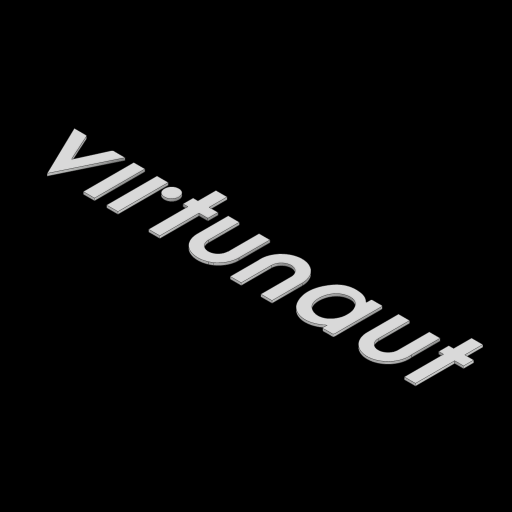
# Autodesk Inventor part: 242_LOGO
Saved by Autodesk Inventor 2024 (Build 280153000, 153)
## iProperties
Created: 2023-07-24
Part Number: 242_LOGO
Material: Generisch
Document SubType Name: Modeling
Designer: Philipp
Density: 1 g/cm^3
Appearance: Vorgabe
Author: Philipp
Autodesk Inventor part; units mm, degrees
ref_plane "YZ Plane" through (0, 0, 0) normal (1, 0, 0) x (0, 1, 0)
ref_plane "XZ Plane" through (0, 0, 0) normal (0, 1, 0) x (-1, 0, 0)
ref_plane "XY Plane" through (0, 0, 0) normal (0, 0, 1) x (1, 0, 0)
sketch "Skizze1" plane through (0, 0, 0) normal (0, 0, 1) x (1, 0, 0)
  line L0 (-37.3972, 3.9318) -> (-43.7451, -9.2055)
  line L1 (-43.7451, -9.2055) -> (-50.0897, 3.9182)
  line L2 (-32.4911, 3.9572) -> (-35.2833, 3.9572)
  line L3 (-35.2833, 3.9572) -> (-35.2833, -8.635)
  line L4 (-35.2833, -8.635) -> (-32.4911, -8.635)
  line L5 (-32.4911, -8.635) -> (-32.4911, 3.9572)
  line L6 (-26.6443, 3.9432) -> (-29.4671, 3.9432)
  line L7 (-29.4671, 3.9432) -> (-29.4671, -8.635)
  line L8 (-29.4671, -8.635) -> (-26.6443, -8.635)
  line L9 (-26.6443, -8.635) -> (-26.6443, 3.9432)
  line L10 (-16.1812, 3.676) -> (-16.1812, 8.1673)
  line L11 (-16.1812, 8.1673) -> (-18.9705, 8.1673)
  line L12 (-18.9705, 8.1673) -> (-18.9705, 3.676)
  line L13 (-18.9705, 3.676) -> (-20.1816, 3.676)
  line L14 (-20.1816, 3.676) -> (-20.1816, 1.149)
  line L15 (-20.1816, 1.149) -> (-18.9705, 1.149)
  line L16 (-18.9705, 1.149) -> (-18.9705, -8.635)
  line L17 (-18.9705, -8.635) -> (-16.1812, -8.635)
  line L18 (-16.1812, -8.635) -> (-16.1812, 1.149)
  line L19 (-16.1812, 1.149) -> (-13.9526, 1.149)
  line L20 (-13.9526, 1.149) -> (-13.9526, 3.676)
  line L21 (-13.9526, 3.676) -> (-16.1812, 3.676)
  arc A0 (-3.6373, -7.7101) -> (-1.5254, -3.5201) centre (-6.7378, -3.5201) ccw
  line L22 (-1.5254, -3.5201) -> (-1.5254, 4.2241)
  line L23 (-1.5254, 4.2241) -> (-4.2557, 4.2241)
  line L24 (-4.2557, 4.2241) -> (-4.2557, -3.5201)
  line L25 (-4.2557, -3.5201) -> (-4.3028, -3.5201)
  arc A1 (-9.1728, -3.5201) -> (-4.3028, -3.5201) centre (-6.7378, -3.5201) ccw
  line L26 (-9.1728, -3.5201) -> (-9.1728, 4.2241)
  line L27 (-9.1728, 4.2241) -> (-11.9502, 4.2241)
  line L28 (-11.9502, 4.2241) -> (-11.9502, -3.5201)
  arc A2 (-11.9502, -3.5201) -> (-10.9081, -6.647) centre (-6.7378, -3.5201) ccw
  line L29 (1.4099, -8.6315) -> (4.1527, -8.6315)
  line L30 (4.1527, -8.6315) -> (4.1527, -1.0852)
  arc A3 (9.0698, -1.0852) -> (4.1527, -1.0852) centre (6.6113, -1.0852) ccw
  line L31 (9.0698, -1.0852) -> (9.0698, -8.6315)
  line L32 (9.0698, -8.6315) -> (11.8472, -8.6315)
  line L33 (11.8472, -8.6315) -> (11.8472, -1.0852)
  arc A4 (11.8472, -1.0852) -> (1.4099, -1.6856) centre (6.6113, -1.0852) ccw
  line L34 (1.4099, -1.6856) -> (1.4099, -8.6315)
  line L35 (33.3608, 4.2241) -> (30.5834, 4.2241)
  line L36 (30.5834, 4.2241) -> (30.5834, -3.6173)
  arc A5 (30.5834, -3.6173) -> (41.0081, -2.916) centre (35.8193, -3.6173) ccw
  line L37 (41.0081, -2.916) -> (41.0081, 4.2241)
  line L38 (41.0081, 4.2241) -> (38.2779, 4.2241)
  line L39 (38.2779, 4.2241) -> (38.2779, -3.6173)
  arc A6 (33.3608, -3.6173) -> (38.2779, -3.6173) centre (35.8193, -3.6173) ccw
  line L40 (33.3608, -3.6173) -> (33.3608, 4.2241)
  line L41 (47.6817, 3.676) -> (47.6817, 8.1673)
  line L42 (47.6817, 8.1673) -> (44.8924, 8.1673)
  line L43 (44.8924, 8.1673) -> (44.8924, 3.676)
  line L44 (44.8924, 3.676) -> (43.6812, 3.676)
  line L45 (43.6812, 3.676) -> (43.6812, 1.149)
  line L46 (43.6812, 1.149) -> (44.8924, 1.149)
  line L47 (44.8924, 1.149) -> (44.8924, -8.635)
  line L48 (44.8924, -8.635) -> (47.6817, -8.635)
  line L49 (47.6817, -8.635) -> (47.6817, 1.149)
  line L50 (47.6817, 1.149) -> (49.9103, 1.149)
  line L51 (49.9103, 1.149) -> (49.9103, 3.676)
  line L52 (49.9103, 3.676) -> (47.6817, 3.676)
  spline S0 degree 3 poles (-50.0897, 3.9182) (-49.0082, 3.9182) (-48.0657, 3.9279) (-47.124, 3.9049) (-47.0171, 3.9023) (-46.8727, 3.7347) (-46.8166, 3.6114) (-45.8869, 1.5682) (-44.9691, -0.4805) (-44.0466, -2.527) (-43.9721, -2.6922) (-43.8826, -2.8505) (-43.7495, -3.1111) knots -10 -10 -10 -10 -9 -9 -9 -8 -8 -8 -7 -7 -7 -6 -6 -6 -6
  line L53 (-50.0897, 3.9182) -> (-49.0082, 3.9182) construction
  line L54 (-49.0082, 3.9182) -> (-48.0657, 3.9279) construction
  line L55 (-48.0657, 3.9279) -> (-47.124, 3.9049) construction
  line L56 (-47.124, 3.9049) -> (-47.0171, 3.9023) construction
  line L57 (-47.0171, 3.9023) -> (-46.8727, 3.7347) construction
  line L58 (-46.8727, 3.7347) -> (-46.8166, 3.6114) construction
  line L59 (-46.8166, 3.6114) -> (-45.8869, 1.5682) construction
  line L60 (-45.8869, 1.5682) -> (-44.9691, -0.4805) construction
  line L61 (-44.9691, -0.4805) -> (-44.0466, -2.527) construction
  line L62 (-44.0466, -2.527) -> (-43.9721, -2.6922) construction
  line L63 (-43.9721, -2.6922) -> (-43.8826, -2.8505) construction
  line L64 (-43.8826, -2.8505) -> (-43.7495, -3.1111) construction
  spline S1 degree 3 poles (-43.7495, -3.1111) (-43.6007, -2.8191) (-43.4873, -2.6166) (-43.3918, -2.406) (-42.4883, -0.4134) (-41.5817, 1.5779) (-40.6937, 3.5774) (-40.5751, 3.8444) (-40.4324, 3.9417) (-40.1479, 3.937) (-39.2783, 3.9226) (-38.4083, 3.9318) (-37.3972, 3.9318) knots -6 -6 -6 -6 -5 -5 -5 -4 -4 -4 -3 -3 -3 -2 -2 -2 -2
  line L65 (-43.7495, -3.1111) -> (-43.6007, -2.8191) construction
  line L66 (-43.6007, -2.8191) -> (-43.4873, -2.6166) construction
  line L67 (-43.4873, -2.6166) -> (-43.3918, -2.406) construction
  line L68 (-43.3918, -2.406) -> (-42.4883, -0.4134) construction
  line L69 (-42.4883, -0.4134) -> (-41.5817, 1.5779) construction
  line L70 (-41.5817, 1.5779) -> (-40.6937, 3.5774) construction
  line L71 (-40.6937, 3.5774) -> (-40.5751, 3.8444) construction
  line L72 (-40.5751, 3.8444) -> (-40.4324, 3.9417) construction
  line L73 (-40.4324, 3.9417) -> (-40.1479, 3.937) construction
  line L74 (-40.1479, 3.937) -> (-39.2783, 3.9226) construction
  line L75 (-39.2783, 3.9226) -> (-38.4083, 3.9318) construction
  line L76 (-38.4083, 3.9318) -> (-37.3972, 3.9318) construction
  line L77 (-35.2833, -8.635) -> (-35.2833, 3.9572)
  line L78 (-32.4911, 3.9572) -> (-32.4911, -8.635)
  spline S2 degree 3 poles (-25.7998, 2.1249) (-25.8047, 3.186) (-25.0538, 3.9433) (-23.9969, 3.9432) (-22.9712, 3.9431) (-22.2131, 3.1845) (-22.2062, 2.1515) (-22.199, 1.0897) (-22.9481, 0.3376) (-24.0112, 0.339) (-25.0478, 0.3403) (-25.7949, 1.0863) (-25.7998, 2.1249) knots -4 -4 -4 -4 -3 -3 -3 -2 -2 -2 -1 -1 -1 0 0 0 0
  line L79 (-25.7998, 2.1249) -> (-25.8047, 3.186) construction
  line L80 (-25.8047, 3.186) -> (-25.0538, 3.9433) construction
  line L81 (-25.0538, 3.9433) -> (-23.9969, 3.9432) construction
  line L82 (-23.9969, 3.9432) -> (-22.9712, 3.9431) construction
  line L83 (-22.9712, 3.9431) -> (-22.2131, 3.1845) construction
  line L84 (-22.2131, 3.1845) -> (-22.2062, 2.1515) construction
  line L85 (-22.2062, 2.1515) -> (-22.199, 1.0897) construction
  line L86 (-22.199, 1.0897) -> (-22.9481, 0.3376) construction
  line L87 (-22.9481, 0.3376) -> (-24.0112, 0.339) construction
  line L88 (-24.0112, 0.339) -> (-25.0478, 0.3403) construction
  line L89 (-25.0478, 0.3403) -> (-25.7949, 1.0863) construction
  line L90 (-25.7949, 1.0863) -> (-25.7998, 2.1249) construction
  spline S3 degree 3 poles (-4.46, -8.156) (-6.479, -9.089) (-9.3621, -8.6813) (-10.9081, -6.647) knots -21 -21 -21 -21 -20.194363 -20.194363 -20.194363 -20.194363
  line L91 (-4.46, -8.156) -> (-6.479, -9.089) construction
  line L92 (-6.479, -9.089) -> (-9.3621, -8.6813) construction
  line L93 (-9.3621, -8.6813) -> (-10.9081, -6.647) construction
  spline S4 degree 3 poles (-3.6373, -7.7101) (-3.8938, -7.8733) (-4.1689, -8.0215) (-4.46, -8.156) knots 0 0 0 0 1 1 1 1
  line L94 (-3.6373, -7.7101) -> (-3.8938, -7.8733) construction
  line L95 (-3.8938, -7.8733) -> (-4.1689, -8.0215) construction
  line L96 (-4.1689, -8.0215) -> (-4.46, -8.156) construction
  spline S5 degree 3 poles (24.221, -2.2151) (24.2468, -1.2347) (24.0056, -0.3451) (23.4565, 0.4672) (22.6198, 1.7049) (21.3436, 2.161) (19.8984, 1.7679) (16.8018, 0.9256) (16.5202, -3.482) (18.2335, -5.0764) (19.907, -6.6338) (22.3784, -6.5552) (23.5807, -4.5663) (24.0246, -3.832) (24.2519, -3.0588) (24.221, -2.2151) knots -5 -5 -5 -5 -4 -4 -4 -3 -3 -3 -2 -2 -2 -1 -1 -1 0 0 0 0
  line L97 (24.221, -2.2151) -> (24.2468, -1.2347) construction
  line L98 (24.2468, -1.2347) -> (24.0056, -0.3451) construction
  line L99 (24.0056, -0.3451) -> (23.4565, 0.4672) construction
  line L100 (23.4565, 0.4672) -> (22.6198, 1.7049) construction
  line L101 (22.6198, 1.7049) -> (21.3436, 2.161) construction
  line L102 (21.3436, 2.161) -> (19.8984, 1.7679) construction
  line L103 (19.8984, 1.7679) -> (16.8018, 0.9256) construction
  line L104 (16.8018, 0.9256) -> (16.5202, -3.482) construction
  line L105 (16.5202, -3.482) -> (18.2335, -5.0764) construction
  line L106 (18.2335, -5.0764) -> (19.907, -6.6338) construction
  line L107 (19.907, -6.6338) -> (22.3784, -6.5552) construction
  line L108 (22.3784, -6.5552) -> (23.5807, -4.5663) construction
  line L109 (23.5807, -4.5663) -> (24.0246, -3.832) construction
  line L110 (24.0246, -3.832) -> (24.2519, -3.0588) construction
  line L111 (24.2519, -3.0588) -> (24.221, -2.2151) construction
  spline S6 degree 3 poles (24.0576, -7.1033) (23.8847, -7.2019) (23.797, -7.2368) (23.7274, -7.2938) (20.9418, -9.578) (16.9957, -8.8788) (15.2913, -5.6975) (13.869, -3.0429) (14.1127, -0.3673) (15.7908, 2.0934) (17.1034, 4.0183) (19.0797, 4.4954) (21.2933, 4.1311) (22.3019, 3.9652) (23.183, 3.504) (23.9158, 2.7678) knots -6 -6 -6 -6 -5 -5 -5 -4 -4 -4 -3 -3 -3 -2 -2 -2 -1 -1 -1 -1
  line L112 (24.0576, -7.1033) -> (23.8847, -7.2019) construction
  line L113 (23.8847, -7.2019) -> (23.797, -7.2368) construction
  line L114 (23.797, -7.2368) -> (23.7274, -7.2938) construction
  line L115 (23.7274, -7.2938) -> (20.9418, -9.578) construction
  line L116 (20.9418, -9.578) -> (16.9957, -8.8788) construction
  line L117 (16.9957, -8.8788) -> (15.2913, -5.6975) construction
  line L118 (15.2913, -5.6975) -> (13.869, -3.0429) construction
  line L119 (13.869, -3.0429) -> (14.1127, -0.3673) construction
  line L120 (14.1127, -0.3673) -> (15.7908, 2.0934) construction
  line L121 (15.7908, 2.0934) -> (17.1034, 4.0183) construction
  line L122 (17.1034, 4.0183) -> (19.0797, 4.4954) construction
  line L123 (19.0797, 4.4954) -> (21.2933, 4.1311) construction
  line L124 (21.2933, 4.1311) -> (22.3019, 3.9652) construction
  line L125 (22.3019, 3.9652) -> (23.183, 3.504) construction
  line L126 (23.183, 3.504) -> (23.9158, 2.7678) construction
  line L127 (23.9158, 2.7678) -> (24.0584, 2.818)
  spline S7 degree 3 poles (24.0584, 2.818) (24.0584, 3.1108) (24.0657, 3.4039) (24.0561, 3.6964) (24.0481, 3.9369) (24.1479, 4.0222) (24.3884, 4.0186) (25.0753, 4.0083) (25.763, 4.0025) (26.4494, 4.0245) (26.7799, 4.0351) (26.8618, 3.9067) (26.8598, 3.5978) (26.8475, 1.694) (26.8502, -0.2099) (26.8499, -2.1139) (26.8495, -4.0177) (26.8402, -5.9217) (26.8613, -7.8253) (26.8655, -8.2121) (26.7497, -8.3182) (26.3761, -8.3005) (25.7476, -8.2708) (25.1158, -8.2701) (24.4873, -8.2989) (24.1311, -8.3153) (24.031, -8.176) (24.0545, -7.854) (24.0706, -7.633) (24.0576, -7.4098) (24.0576, -7.1033) knots -16 -16 -16 -16 -15 -15 -15 -14 -14 -14 -13 -13 -13 -12 -12 -12 -11 -11 -11 -10 -10 -10 -9 -9 -9 -8 -8 -8 -7 -7 -7 -6 -6 -6 -6
  line L128 (24.0584, 2.818) -> (24.0584, 3.1108) construction
  line L129 (24.0584, 3.1108) -> (24.0657, 3.4039) construction
  line L130 (24.0657, 3.4039) -> (24.0561, 3.6964) construction
  line L131 (24.0561, 3.6964) -> (24.0481, 3.9369) construction
  line L132 (24.0481, 3.9369) -> (24.1479, 4.0222) construction
  line L133 (24.1479, 4.0222) -> (24.3884, 4.0186) construction
  line L134 (24.3884, 4.0186) -> (25.0753, 4.0083) construction
  line L135 (25.0753, 4.0083) -> (25.763, 4.0025) construction
  line L136 (25.763, 4.0025) -> (26.4494, 4.0245) construction
  line L137 (26.4494, 4.0245) -> (26.7799, 4.0351) construction
  line L138 (26.7799, 4.0351) -> (26.8618, 3.9067) construction
  line L139 (26.8618, 3.9067) -> (26.8598, 3.5978) construction
  line L140 (26.8598, 3.5978) -> (26.8475, 1.694) construction
  line L141 (26.8475, 1.694) -> (26.8502, -0.2099) construction
  line L142 (26.8502, -0.2099) -> (26.8499, -2.1139) construction
  line L143 (26.8499, -2.1139) -> (26.8495, -4.0177) construction
  line L144 (26.8495, -4.0177) -> (26.8402, -5.9217) construction
  line L145 (26.8402, -5.9217) -> (26.8613, -7.8253) construction
  line L146 (26.8613, -7.8253) -> (26.8655, -8.2121) construction
  line L147 (26.8655, -8.2121) -> (26.7497, -8.3182) construction
  line L148 (26.7497, -8.3182) -> (26.3761, -8.3005) construction
  line L149 (26.3761, -8.3005) -> (25.7476, -8.2708) construction
  line L150 (25.7476, -8.2708) -> (25.1158, -8.2701) construction
  line L151 (25.1158, -8.2701) -> (24.4873, -8.2989) construction
  line L152 (24.4873, -8.2989) -> (24.1311, -8.3153) construction
  line L153 (24.1311, -8.3153) -> (24.031, -8.176) construction
  line L154 (24.031, -8.176) -> (24.0545, -7.854) construction
  line L155 (24.0545, -7.854) -> (24.0706, -7.633) construction
  line L156 (24.0706, -7.633) -> (24.0576, -7.4098) construction
  line L157 (24.0576, -7.4098) -> (24.0576, -7.1033) construction
  point P0 (0, 0)
  point P1 (41.0081, -2.916)
  point P2 (23.9158, 2.7678)
  point P3 (1.4099, -1.6856)
  point P4 (4.1527, -8.6315)
  point P5 (-4.4592, -8.1556)
  point P6 (-3.6373, -7.7101)
  point P7 (-1.5254, -3.5201)
  point P8 (-9.1728, -3.5201)
  point P9 (-11.9502, -3.5201)
  point P10 (-10.9061, -6.6496)
  point P11 (-32.4911, 3.9572)
  point P12 (-37.3978, 3.9305)
  point P13 (-50.0897, 3.9182)
  constraints: 112 end point, 14 point on circle, 7 centre point, 22 other
extrude "Extrusion1" add sketch "Skizze1" along normal blind 0.6
